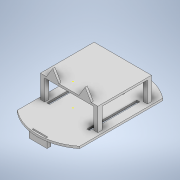
# Autodesk Inventor part: rinetracer1
Saved by Autodesk Inventor 2021.1 (Build 251245010, 245A)
## iProperties
Created: 2021-01-30
Part Number: rinetracer1
Material: Generic
Document SubType Name: Modeling
Designer: User
Density: 1 g/cm^3
Appearance: Default
Author: User
Autodesk Inventor part; units mm, degrees
ref_plane "YZ Plane" through (0, 0, 0) normal (1, 0, 0) x (0, 1, 0)
ref_plane "XZ Plane" through (0, 0, 0) normal (0, 1, 0) x (-1, 0, 0)
ref_plane "XY Plane" through (0, 0, 0) normal (0, 0, 1) x (1, 0, 0)
sketch "스케치1" plane through (0, 0, 0) normal (0, 1, 0) x (-1, 0, 0)
  line L0 (-87.543698, 71.443249) -> (-87.543698, -128.556751)
  line L1 (62.456302, -128.556751) -> (62.456302, 71.443249)
  arc A0 (-87.543698, -128.556751) -> (62.456302, -128.556751) centre (-12.543698, -33.887174) ccw
  arc A1 (62.456302, 71.443249) -> (-87.543698, 71.443249) centre (-12.543698, -23.226328) ccw
  line L2 (62.456302, 71.443249) -> (-87.543698, 71.443249)
  line L3 (62.456302, -128.556751) -> (-87.543698, -128.556751)
  line L4 (15.552801, 94.238201) -> (-36.133127, 94.238201)
  line L5 (-36.133127, 94.238201) -> (-36.133127, 84.238201)
  line L6 (-36.133127, 84.238201) -> (15.552801, 84.238201)
  line L7 (15.552801, 84.238201) -> (15.552801, 94.238201)
  line L8 (52.977173, -113.513448) -> (42.977173, -113.513448)
  line L9 (42.977173, -113.513448) -> (42.977173, -103.513448)
  line L10 (42.977173, -103.513448) -> (52.977173, -103.513448)
  line L11 (52.977173, -103.513448) -> (52.977173, -113.513448)
  line L12 (-65.755771, -113.513448) -> (-75.755771, -113.513448)
  line L13 (-75.755771, -113.513448) -> (-75.755771, -103.513448)
  line L14 (-75.755771, -103.513448) -> (-65.755771, -103.513448)
  line L15 (-65.755771, -103.513448) -> (-65.755771, -113.513448)
  line L16 (52.977173, 47.521121) -> (42.977173, 47.521121)
  line L17 (42.977173, 47.521121) -> (42.977173, 57.521121)
  line L18 (42.977173, 57.521121) -> (52.977173, 57.521121)
  line L19 (52.977173, 57.521121) -> (52.977173, 47.521121)
  line L20 (-65.082073, 47.521121) -> (-75.082073, 47.521121)
  line L21 (-75.082073, 57.521121) -> (-65.082073, 57.521121)
  line L22 (-75.082073, 47.521121) -> (-75.082073, 57.521121)
  line L23 (-65.082073, 57.521121) -> (-65.082073, 47.521121)
  point P0 (0, 0)
  dimension "d4" = 150
  dimension "d5" = 200
  dimension "d6" = 10
  dimension "d12" = 10
  dimension "d13" = 10
  dimension "d20" = 10
  dimension "d21" = 10
  dimension "d22" = 10
  dimension "d23" = 10
  dimension "d24" = 10
  dimension "d25" = 10
  constraints: 48 end point, 12 parallel, 6 horizontal, 5 perpendicular, 5 point on circle, 2 centre point, 1 equal radius
  measures "d4" distance between parallel lines of L0 L1
  measures "d5" distance between parallel lines of L3 L2
  measures "d6" distance between parallel lines of L6 L4
  measures "d12" distance between parallel lines of L9 L11
  measures "d13" distance between parallel lines of L10 L8
  measures "d20" distance between parallel lines of L13 L15
  measures "d21" distance between parallel lines of L14 L12
  measures "d22" distance between parallel lines of L17 L19
  measures "d23" distance between parallel lines of L18 L16
  measures "d24" distance between parallel lines of L22 L23
  measures "d25" distance between parallel lines of L21 L20
sketch "스케치1 outline for 돌출1" plane through (0, 0, 0) normal (0, 1, 0) x (-1, 0, 0)
  arc A0 (62.456302, 71.443249) -> (-87.543698, 71.443249) centre (-12.543698, -23.226328) ccw
  line L0 (62.456302, -128.556751) -> (62.456302, 71.443249)
  arc A1 (-87.543698, -128.556751) -> (62.456302, -128.556751) centre (-12.543698, -33.887174) ccw
  line L1 (-87.543698, 71.443249) -> (-87.543698, -128.556751)
extrude "돌출1" add sketch "스케치1 outline for 돌출1" along normal blind 5
sketch "스케치3" plane through (0, 5, 0) normal (0, 1, 0) x (1, 0, 0)
  arc A0 (-62.456302, -71.443249) -> (87.543698, -71.443249) centre (12.543698, 23.226328) ccw
  line L0 (-10.169389, -95.396792) -> (33.095027, -95.396792)
  line L1 (33.095027, -95.396792) -> (33.095027, -86.258943)
  line L2 (33.095027, -86.258943) -> (-10.169389, -86.258943)
  line L3 (-10.169389, -86.258943) -> (-10.169389, -95.396792)
  point P0 (0, 0)
  constraints: 8 end point, 2 parallel, 1 horizontal, 1 perpendicular, 1 point on circle
extrude "돌출2" add sketch "스케치3" against normal blind 20
sketch "스케치4" plane through (0, 5, 0) normal (0, 1, 0) x (1, 0, 0)
  line L0 (-56.990746, -11.07401) -> (-46.990746, -11.07401)
  line L1 (-46.990746, -11.07401) -> (-46.990746, -21.07401)
  line L2 (-46.990746, -21.07401) -> (-56.990746, -21.07401)
  line L3 (-56.990746, -21.07401) -> (-56.990746, -11.07401)
  line L4 (-56.990746, 107.98138) -> (-46.990746, 107.98138)
  line L5 (-46.990746, 107.98138) -> (-46.990746, 97.98138)
  line L6 (-46.990746, 97.98138) -> (-56.990746, 97.98138)
  line L7 (-56.990746, 97.98138) -> (-56.990746, 107.98138)
  line L8 (71.101861, -11.07401) -> (81.101861, -11.07401)
  line L9 (81.101861, -11.07401) -> (81.101861, -21.07401)
  line L10 (81.101861, -21.07401) -> (71.101861, -21.07401)
  line L11 (71.101861, -21.07401) -> (71.101861, -11.07401)
  line L12 (71.101861, 108.118279) -> (81.101861, 108.118279)
  line L13 (81.101861, 98.118279) -> (71.101861, 98.118279)
  line L14 (81.101861, 108.118279) -> (81.101861, 98.118279)
  line L15 (71.101861, 98.118279) -> (71.101861, 108.118279)
  point P0 (0, 0)
  dimension "d31" = 10
  dimension "d32" = 10
  dimension "d33" = 10
  dimension "d34" = 10
  dimension "d35" = 10
  dimension "d36" = 10
  dimension "d37" = 10
  dimension "d38" = 10
  constraints: 32 end point, 8 parallel, 4 horizontal, 4 perpendicular
  measures "d31" distance between parallel lines of L2 L0
  measures "d32" distance between parallel lines of L1 L3
  measures "d33" distance between parallel lines of L6 L4
  measures "d34" distance between parallel lines of L5 L7
  measures "d35" distance between parallel lines of L10 L8
  measures "d36" distance between parallel lines of L9 L11
  measures "d37" distance between parallel lines of L13 L12
  measures "d38" distance between parallel lines of L14 L15
extrude "돌출3" add sketch "스케치4" along normal blind 50
sketch "스케치5" plane through (0, 55, 0) normal (0, 1, 0) x (1, 0, 0)
  line L0 (-46.990746, 107.98138) -> (-56.990746, 107.98138)
  line L1 (71.101861, -21.07401) -> (81.101861, -21.07401)
  line L2 (-56.990746, 107.98138) -> (81.101861, 107.98138)
  line L3 (81.101861, 107.98138) -> (81.101861, -21.07401)
  line L4 (81.101861, -21.07401) -> (-56.990746, -21.07401)
  line L5 (-56.990746, -21.07401) -> (-56.990746, 107.98138)
  point P0 (0, 0)
  constraints: 8 end point, 2 parallel, 1 horizontal, 1 perpendicular
extrude "돌출4" add sketch "스케치5" along normal blind 5
sketch "스케치6" plane through (0, 60, 0) normal (0, 1, 0) x (1, 0, 0)
  point P0 (0, 0)
sketch "스케치7" plane through (71.101861, 5, 21.07401) normal (0, 0, 1) x (1, 0, 0)
  line L0 (-128.092607, 55) -> (10, 55)
  line L1 (-113.361427, 55) -> (-98.565379, 79.478069)
  line L2 (-98.565379, 79.478069) -> (-83.769331, 55)
  line L3 (-35.573927, 55) -> (-20.777879, 79.478069)
  line L4 (-20.777879, 79.478069) -> (-5.981831, 55)
  point P0 (-71.101861, -5)
  constraints: 8 end point, 2 equal length, 2 point on line
extrude "돌출5" add sketch "스케치7" against normal blind 5
sketch "스케치8" plane through (81.101861, 5, -108.118279) normal (0, 0, -1) x (-1, 0, 0)
  point P0 (81.101861, -5)
sketch "스케치9" plane through (0, 5, 0) normal (0, 1, 0) x (1, 0, 0)
  point P0 (0, 0)
sketch "스케치10" plane through (0, 5, 0) normal (0, 1, 0) x (1, 0, 0)
  line L0 (60.543698, -26.9875) -> (67.543698, -26.9875)
  line L1 (67.543698, -26.9875) -> (67.543698, 93.6625)
  line L2 (67.543698, 93.6625) -> (60.543698, 93.6625)
  line L3 (60.543698, 93.6625) -> (60.543698, -26.9875)
  line L4 (87.543698, -71.443249) -> (87.543698, 128.556751)
  line L5 (-42.456302, -20.6375) -> (-35.456302, -20.6375)
  line L6 (-35.456302, -20.6375) -> (-35.456302, 100.0125)
  line L7 (-35.456302, 100.0125) -> (-42.456302, 100.0125)
  line L8 (-42.456302, 100.0125) -> (-42.456302, -20.6375)
  line L9 (-62.456302, 128.556751) -> (-62.456302, -71.443249)
  circle A0 centre (-2.456302, 90.4875) radius 4.490128
  circle A1 centre (27.543698, 90.4875) radius 4.490128
  circle A2 centre (26.784766, 120.477899) radius 4.490128
  circle A3 centre (-3.215233, 120.4875) radius 4.490128
  point P0 (0, 0)
  dimension "d45" = 20
  dimension "d46" = 7
  dimension "d47" = 7
  dimension "d48" = 20
  dimension "d53" = 30
  dimension "d54" = 60
  dimension "d55" = 30
  dimension "d56" = 30
  dimension "d57" = 30
  constraints: 16 end point, 4 centre point, 4 parallel, 2 horizontal, 2 perpendicular
  measures "d45" distance between parallel lines of L4 L1
  measures "d46" distance between parallel lines of L1 L3
  measures "d47" distance between parallel lines of L6 L8
  measures "d48" distance between parallel lines of L9 L8
  measures "d53" distance of A0.centre A1.centre
  measures "d54" distance from line of A1.centre L4
  measures "d55" distance of A2.centre A1.centre
  measures "d56" vertical distance of A3.centre A0.centre
  measures "d57" distance of A3.centre A2.centre
extrude "돌출6" cut sketch "스케치10" against normal blind 10
sketch "스케치11" plane through (0, 5, 0) normal (0, 1, 0) x (1, 0, 0)
  point P0 (0, 0)
sketch "스케치14" plane through (0, 5, 0) normal (0, 1, 0) x (1, 0, 0)
  line L0 (-4.7625, -90.4875) -> (30.1625, -90.4875)
  line L1 (30.1625, -90.4875) -> (30.1625, -93.6625)
  line L2 (30.1625, -93.6625) -> (-4.7625, -93.6625)
  line L3 (-4.7625, -93.6625) -> (-4.7625, -90.4875)
  point P0 (0, 0)
  constraints: 8 end point, 2 parallel, 1 horizontal, 1 perpendicular
extrude "돌출8" cut sketch "스케치14" against normal blind 30
